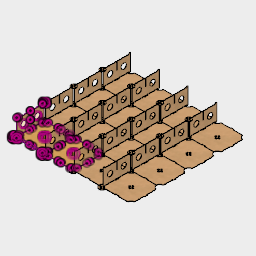
Mirobot_Labyrinth (Autodesk Fusion 360 design; units mm, degrees)
Autodesk Fusion 360 part; units mm, degrees
sketch "Sketch1" plane through (0, 0, 0) normal (0, 1, 0) x (1, 0, 0)
  line L0 (251.5519, -328.5135) -> (251.5519, -318.5135)
  line L1 (251.5519, -318.5135) -> (246.5519, -318.5135)
  line L2 (251.5519, -148.5135) -> (251.5519, -158.5135)
  line L3 (251.5519, -158.5135) -> (246.5519, -158.5135)
  line L4 (140.5519, -148.5135) -> (140.5519, -158.5135)
  line L5 (140.5519, -158.5135) -> (146.5519, -158.5135)
  line L6 (140.5519, -328.5135) -> (140.5519, -318.5135)
  line L7 (146.5519, -318.5135) -> (140.5519, -318.5135)
  line L8 (146.5519, -158.5135) -> (146.5519, -237.0135)
  line L9 (246.5519, -318.5135) -> (246.5519, -158.5135)
  circle A0 centre (166.0327, -110.4808) radius 17.5
  line L10 (251.5519, -328.5135) -> (140.5519, -328.5135)
  line L11 (140.5519, -148.5135) -> (251.5519, -148.5135)
  line L12 (161.0327, -108.9808) -> (161.0327, -111.9808)
  line L13 (161.0327, -111.9808) -> (151.0327, -111.9808)
  line L14 (151.0327, -111.9808) -> (151.0327, -108.9808)
  line L15 (151.0327, -108.9808) -> (161.0327, -108.9808)
  line L16 (167.5327, -125.4808) -> (164.5327, -125.4808)
  line L17 (164.5327, -125.4808) -> (164.5327, -115.4808)
  line L18 (167.5327, -115.4808) -> (167.5327, -125.4808)
  line L19 (164.5327, -115.4808) -> (167.5327, -115.4808)
  line L20 (181.0327, -108.9808) -> (181.0327, -111.9808)
  line L21 (181.0327, -111.9808) -> (171.0327, -111.9808)
  line L22 (171.0327, -108.9808) -> (181.0327, -108.9808)
  line L23 (171.0327, -111.9808) -> (171.0327, -108.9808)
  line L24 (164.5327, -95.4808) -> (167.5327, -95.4808)
  line L25 (167.5327, -95.4808) -> (167.5327, -105.4808)
  line L26 (164.5327, -105.4808) -> (164.5327, -95.4808)
  line L27 (167.5327, -105.4808) -> (164.5327, -105.4808)
  circle A1 centre (473.7067, -121) radius 5.0194
  circle A2 centre (463.7296, -110.8358) radius 5
  circle A3 centre (453.7523, -121) radius 5
  circle A4 centre (463.7296, -130.8358) radius 5
  circle A5 centre (663.7067, -121) radius 5.0194
  circle A6 centre (653.7296, -110.8358) radius 5
  circle A7 centre (643.7523, -121) radius 5
  circle A8 centre (653.7296, -130.8358) radius 5
  circle A9 centre (473.7067, 69) radius 5.0194
  circle A10 centre (463.7296, 79.1642) radius 5
  circle A11 centre (453.7523, 69) radius 5
  circle A12 centre (463.7296, 59.1642) radius 5
  circle A13 centre (663.7067, 69) radius 5.0194
  circle A14 centre (653.7296, 79.1642) radius 5
  circle A15 centre (643.7523, 69) radius 5
  circle A16 centre (653.7296, 59.1642) radius 5
  line L28 (443.2442, 139.3735) -> (443.2442, 139.3735)
  line L29 (436.89, 127.8892) -> (266.89, 127.8892)
  line L30 (259.39, 135.3765) -> (259.39, 135.3765)
  line L31 (266.89, 142.8892) -> (436.89, 142.8892)
  circle A17 centre (436.89, 135.3892) radius 5
  arc A18 (266.89, 142.8892) -> (259.39, 135.3765) centre (266.89, 135.3892) ccw
  arc A19 (259.39, 135.3765) -> (266.89, 127.8892) centre (266.89, 135.3892) ccw
  circle A20 centre (266.89, 135.3892) radius 5
  line L32 (453.7523, -121) -> (473.7067, -121) construction
  line L33 (463.7296, -110.8358) -> (463.7296, -130.8358) construction
  circle A21 centre (463.7295, -121) radius 25 construction
  line L34 (463.7295, -121) -> (463.7295, -146) construction
  line L35 (463.7295, -121) -> (488.7295, -121) construction
  line L36 (463.7295, -121) -> (438.7295, -121) construction
  line L37 (463.7295, -121) -> (463.7295, -96) construction
  line L38 (643.7523, -121) -> (663.7067, -121) construction
  line L39 (653.7296, -110.8358) -> (653.7296, -130.8358) construction
  circle A22 centre (653.7295, -121) radius 25 construction
  line L40 (453.7523, 69) -> (473.7067, 69) construction
  line L41 (463.7296, 79.1642) -> (463.7296, 59.1642) construction
  circle A23 centre (463.7295, 69) radius 25 construction
  line L42 (643.7523, 69) -> (663.7067, 69) construction
  line L43 (653.7296, 59.1642) -> (653.7296, 79.1642) construction
  circle A24 centre (653.7296, 69.1642) radius 25 construction
  line L44 (457.4795, -102.25) -> (461.2974, -102.25) construction
  line L45 (444.9795, -114.75) -> (449.7421, -114.75) construction
  line L46 (444.9795, -127.25) -> (440.1499, -128.5441)
  line L47 (456.1854, -144.5796) -> (440.1499, -128.5441)
  line L48 (457.4795, -139.75) -> (456.1854, -144.5796)
  line L49 (469.9795, -139.75) -> (471.2736, -144.5796)
  line L50 (487.3091, -128.5441) -> (471.2736, -144.5796)
  line L51 (482.4795, -127.25) -> (487.3091, -128.5441)
  line L52 (647.4795, -102.25) -> (646.1854, -97.4204)
  line L53 (630.1499, -113.4559) -> (646.1854, -97.4204)
  line L54 (634.9795, -114.75) -> (630.1499, -113.4559)
  line L55 (634.9795, -114.75) -> (628.7295, -121)
  line L56 (647.4799, 50.25) -> (646.1858, 45.4204)
  line L57 (646.1858, 45.4204) -> (630.1503, 61.4559)
  line L58 (634.9799, 62.75) -> (630.1503, 61.4559)
  line L59 (440.1499, -113.4559) -> (456.1854, -97.4204)
  line L60 (487.3091, 61.4559) -> (471.2736, 45.4204)
  line L61 (482.4795, 62.75) -> (487.3091, 61.4559)
  line L62 (482.4795, 62.75) -> (488.7295, 69)
  line L63 (469.9795, 50.25) -> (471.2736, 45.4204)
  line L64 (463.7293, -17.1612) -> (463.7295, 44)
  line L65 (463.7293, -17.1612) -> (468.0594, -14.6612)
  line L66 (468.0594, -14.6612) -> (468.0594, -37.3388)
  line L67 (463.7293, -34.8388) -> (468.0594, -37.3388)
  line L68 (463.7293, -34.8388) -> (463.729, -96)
  line L69 (653.7293, -34.8388) -> (653.729, -96)
  line L70 (653.7293, -34.8388) -> (658.0594, -37.3388)
  line L71 (658.0594, -14.6612) -> (658.0594, -37.3388)
  line L72 (653.7293, -17.1612) -> (658.0594, -14.6612)
  line L73 (653.7293, -17.1612) -> (653.7295, 44)
  line L74 (567.5683, -121.0002) -> (570.0683, -116.6701)
  line L75 (547.3907, -116.6701) -> (570.0683, -116.6701)
  line L76 (549.8907, -121.0002) -> (547.3907, -116.6701)
  line L77 (567.5683, 68.9998) -> (628.7295, 68.9996)
  line L78 (547.3907, 73.3299) -> (570.0683, 73.3299)
  line L79 (549.8907, 68.9998) -> (547.3907, 73.3299)
  line L80 (567.5683, 68.9998) -> (570.0683, 73.3299)
  line L81 (549.8907, 68.9998) -> (488.7295, 69)
  line L82 (628.7295, -121) -> (567.5683, -121.0002)
  line L83 (549.8907, -121.0002) -> (488.7295, -121)
  line L84 (469.9795, -139.75) -> (463.7295, -146)
  line L85 (482.4795, -127.25) -> (488.7295, -121)
  line L86 (457.4795, -139.75) -> (463.7295, -146)
  line L87 (444.9795, -127.25) -> (438.7295, -121)
  line L88 (438.7295, -121) -> (444.9795, -114.75)
  line L89 (444.9795, -114.75) -> (440.1499, -113.4559)
  line L90 (457.4795, -102.25) -> (456.1854, -97.4204)
  line L91 (463.729, -96) -> (457.4795, -102.25)
  line L92 (463.7295, 44) -> (469.9795, 50.25)
  line L93 (634.9799, 62.75) -> (628.7295, 68.9996)
  line L94 (653.7295, 44) -> (647.4799, 50.25)
  line L95 (653.729, -96) -> (647.4795, -102.25)
  arc A25 (436.89, 127.8892) -> (436.89, 142.8892) centre (436.89, 135.3892) ccw
  line L96 (146.5519, -240.0135) -> (146.5519, -318.5135)
  line L97 (196.5519, -240.0135) -> (146.5519, -240.0135)
  line L98 (196.5519, -237.0135) -> (146.5519, -237.0135)
  line L99 (196.5519, -237.0135) -> (196.5519, -240.0135)
  line L100 (198.0519, -178.5135) -> (198.0519, -188.5135)
  line L101 (195.0519, -188.5135) -> (195.0519, -178.5135)
  line L102 (191.5519, -192.0135) -> (191.5519, -195.0135)
  line L103 (211.5519, -192.0135) -> (211.5519, -195.0135)
  line L104 (191.5519, -195.0135) -> (181.5519, -195.0135)
  line L105 (195.0519, -208.5135) -> (195.0519, -198.5135)
  line L106 (198.0519, -198.5135) -> (198.0519, -208.5135)
  line L107 (198.0519, -208.5135) -> (195.0519, -208.5135)
  circle A26 centre (196.5519, -193.5135) radius 17.5
  line L108 (181.5519, -195.0135) -> (181.5519, -192.0135)
  line L109 (195.0519, -198.5135) -> (198.0519, -198.5135)
  line L110 (195.0519, -178.5135) -> (198.0519, -178.5135)
  line L111 (211.5519, -195.0135) -> (201.5519, -195.0135)
  line L112 (181.5519, -192.0135) -> (191.5519, -192.0135)
  line L113 (201.5519, -195.0135) -> (201.5519, -192.0135)
  line L114 (198.0519, -188.5135) -> (195.0519, -188.5135)
  line L115 (201.5519, -192.0135) -> (211.5519, -192.0135)
  line L116 (246.5519, -238.5135) -> (146.5519, -238.5135) construction
  circle A27 centre (196.5519, -283.5135) radius 17.5
  line L117 (201.5519, -285.0135) -> (211.5519, -285.0135)
  line L118 (211.5519, -285.0135) -> (211.5519, -282.0135)
  line L119 (201.5519, -282.0135) -> (201.5519, -285.0135)
  line L120 (211.5519, -282.0135) -> (201.5519, -282.0135)
  line L121 (195.0519, -298.5135) -> (198.0519, -298.5135)
  line L122 (198.0519, -298.5135) -> (198.0519, -288.5135)
  line L123 (195.0519, -288.5135) -> (195.0519, -298.5135)
  line L124 (198.0519, -288.5135) -> (195.0519, -288.5135)
  line L125 (181.5519, -282.0135) -> (181.5519, -285.0135)
  line L126 (181.5519, -285.0135) -> (191.5519, -285.0135)
  line L127 (191.5519, -282.0135) -> (181.5519, -282.0135)
  line L128 (191.5519, -285.0135) -> (191.5519, -282.0135)
  line L129 (198.0519, -268.5135) -> (195.0519, -268.5135)
  line L130 (195.0519, -268.5135) -> (195.0519, -278.5135)
  line L131 (198.0519, -278.5135) -> (198.0519, -268.5135)
  line L132 (195.0519, -278.5135) -> (198.0519, -278.5135)
  line L133 (463.7295, -121) -> (653.7296, 69.1642) construction
  line L134 (653.7295, -121) -> (463.7295, 69) construction
  circle A28 centre (568.7067, -26) radius 5.0194
  circle A29 centre (558.7296, -35.8358) radius 5
  circle A30 centre (548.7523, -26) radius 5
  circle A31 centre (558.7296, -15.8358) radius 5
  dimension "d4" = 10
  dimension "d6" = 10
  dimension "d7" = 10
  dimension "d8" = 3
  dimension "d11" = 180
  dimension "d12" = 100
  dimension "d34" = 5
  dimension "d50" = 10
  dimension "d53" = 10
  dimension "d66" = 6
  dimension "d80" = 50
  dimension "d83" = 50
  dimension "d85" = 50
  dimension "d87" = 50
  dimension "d109" = 170
  dimension "d113" = 170
  dimension "d124" = 111
  constraint perpendicular L12 L13
  constraint parallel L12 L14
  constraint parallel L13 L15
  constraint tangent L31 A18
  constraint tangent L29 A19
  constraint concentric A19 A20
  constraint horizontal L32
  constraint vertical L33
  constraint midpoint L32
  constraint coincident A21
  constraint perpendicular L32 L34
  constraint coincident A21 origin
  constraint perpendicular L33 L35
  constraint parallel L32 L36
  constraint parallel L33 L37
  constraint horizontal L38
  constraint midpoint L38
  constraint horizontal L40
  constraint perpendicular L40 L41
  constraint midpoint L40
  constraint horizontal L42
  constraint midpoint L43
  constraint horizontal L44
  constraint horizontal L45
  constraint perpendicular L84 L86
  constraint perpendicular L87 L88
  constraint vertical L9
  constraint horizontal L10
  constraint vertical L0
  constraint vertical L2
  constraint horizontal L3
  constraint horizontal L5
  constraint collinear L3 L5
  constraint collinear L1 L7
  constraint horizontal L29
  constraint perpendicular L96 L97
  constraint perpendicular L8 L98
  constraint perpendicular L97 L99
  constraint midpoint L9
  constraint perpendicular L9 L116
  constraint midpoint L134 origin
  measures "d11" distance of L10 L11
  measures "d12" distance of L8 L9
  measures "d50" diameter of A17
  measures "d53" diameter of A20
  measures "d66" distance of L4 L8
  measures "d80" diameter of A21
  measures "d83" diameter of A22
  measures "d85" diameter of A23
  measures "d87" diameter of A24
extrude "Extrude1" add sketch "Sketch1" along normal blind 3 contours L0 L1 L2 L3 L4 L5 L6 L7 L8 L9 L10 L11 L96 L97 L98 L99 | A0 | L29 L31 A18 A19 A25 | L46 L47 L48 L49 L50 L51 L52 L53 L54 L55 L56 L57 L58 L59 L60 L61 L62 L63 L64 L65 L66 L67 L68 L69 L70 L71 L72 L73 L74 L75 L76 L77 L78 L79 L80 L81 L82 L83 L84 L85 L86 L87 L88 L89 L90 L91 L92 L93 L94 L95 makes body 1 at (169.9494, 0, 122.1993) makes body 2 at (235.7186, 0, 223.5135) makes body 3 at (624.1003, 0, 53.8911) makes body 4 at (379.0016, 0, -129.2555)
move_body "MoveBody1" bodies 3 to x (1, 0, 0) y (0, 1, 0) z (0, 0, 1) at (-82.5386, 0, 153.1726)
pattern_linear "R-Pattern1" count 4 spacing 190 along (1, 0, 0) count 4 spacing 190 along (0, 0, -1) of bodies 3 makes body 5 at (731.5617, 0, 207.0637) makes body 6 at (921.5617, 0, 207.0637) makes body 7 at (1111.5617, 0, 207.0637) makes body 8 at (541.5617, 0, 17.0637) makes body 9 at (731.5617, 0, 17.0637) makes body 10 at (921.5617, 0, 17.0637) makes body 11 at (1111.5617, 0, 17.0637) makes body 12 at (541.5617, 0, -172.9363) makes body 13 at (731.5617, 0, -172.9363) makes body 14 at (921.5617, 0, -172.9363) makes body 15 at (1111.5617, 0, -172.9363) makes body 16 at (541.5617, 0, -362.9363) makes body 17 at (731.5617, 0, -362.9363) makes body 18 at (921.5617, 0, -362.9363) makes body 19 at (1111.5617, 0, -362.9363)
move_body "MoveBody2" bodies 4 to x (1, 0, 0) y (0, 1, 0) z (0, 0, 1) at (132.574, 0, 554.7873)
move_body "MoveBody3" bodies 2 to x (0, 1, 0) y (-1, 0, 0) z (0, 0, 1) at (253.0519, -248.5519, 0)
move_body "MoveBody4" bodies 2 to x (1, 0, 0) y (0, 0, 1) z (0, -1, 0) at (141.1162, 321.5135, 380.1726)
move_body "MoveBody5" bodies 2 to x (1, 0, 0) y (0, 0, -1) z (0, 1, 0) at (0, -271.1726, 457.1726)
move_body "MoveBody6" bodies 2 to x (1, 0, 0) y (0, 1, 0) z (0, 0, 1) at (-10.6592, 0, -193.683)
move_body "MoveBody7" bodies 2 to x (1, 0, 0) y (0, -1, 0) z (0, 0, -1) at (-1, 112, 338.9791)
move_body "MoveBody8" bodies 2 to x (1, 0, 0) y (0, 1, 0) z (0, 0, 1) at (0, 0, 20)
move_body "MoveBody9" bodies 2 to x (1, 0, 0.000003) y (0, 1, 0) z (-0.000003, 0, 1) at (1.6823, 0, -0.0013)
move_body "MoveBody10" bodies 2 to x (1, 0, 0) y (0, 1, 0) z (0, 0, 1) at (0, 0, 5.6829)
move_body "MoveBody11" bodies 2 to x (1, 0, 0) y (0, 1, 0) z (0, 0, 1) at (0, 0, -5.164)
move_body "MoveBody12" bodies 2 to x (1, 0, 0) y (0, 1, 0) z (0, 0, 1) at (-1.5, 0, 0)
pattern_linear "R-Pattern2" count 4 spacing 190 along (0, 0, -1) count 4 spacing 190 along (1, 0, 0) of bodies 2 makes body 20 at (382.6907, 15.8333, -25.9915) makes body 21 at (382.6907, 15.8333, -215.9915) makes body 22 at (382.6907, 15.8333, -405.9915) makes body 23 at (572.6907, 15.8333, 164.0085) makes body 24 at (572.6907, 15.8333, -25.9915) makes body 25 at (572.6907, 15.8333, -215.9915) makes body 26 at (572.6907, 15.8333, -405.9915) makes body 27 at (762.6907, 15.8333, 164.0085) makes body 28 at (762.6907, 15.8333, -25.9915) makes body 29 at (762.6907, 15.8333, -215.9915) makes body 30 at (762.6907, 15.8333, -405.9915) makes body 31 at (952.6907, 15.8333, 164.0085) makes body 32 at (952.6907, 15.8333, -25.9915) makes body 33 at (952.6907, 15.8333, -215.9915) makes body 34 at (952.6907, 15.8333, -405.9915)
move_body "MoveBody13" bodies 4 to x (1, 0, 0) y (0, 1, 0) z (0, 0, 1) at (-8.2959, 3, -145.2256)
sketch "Sketch3" plane through (0, 0, 0) normal (0, 1, 0) x (1, 0, 0)
  line L0 (50, -100) -> (50, -94)
  line L1 (50, -94) -> (60, -94)
  line L2 (60, -94) -> (60, -100)
  line L3 (60, -100) -> (63, -100)
  line L4 (63, -100) -> (63, -103)
  line L5 (63, -103) -> (47, -103)
  line L6 (47, -103) -> (47, -100)
  line L7 (47, -100) -> (50, -100)
  dimension "d114" = 3
  dimension "d115" = 3
  dimension "d116" = 16
  constraint horizontal L5
  constraint vertical L4
  constraint horizontal L3
  constraint vertical L2
  constraint vertical L0
  constraint horizontal L7
  constraint horizontal L1
  constraint vertical L6
extrude "Extrude2" add sketch "Sketch3" along normal blind 3 separate body makes body 35
move_body "MoveBody14" bodies 35 to x (1, 0, 0) y (0, 1, 0) z (0, 0, 1) at (349.6709, 0, 195.1812)
move_body "MoveBody15" bodies 35 to x (1, 0, 0) y (0, 0, -1) z (0, 1, 0) at (-13.5028, -289.1812, 275.6726)
move_body "MoveBody16" bodies 1 to x (1, 0, 0.000003) y (0.000003, 0, -1) z (0, 1, 0) at (203.6582, -2.9808, 97.0079)
move_body "MoveBody17" bodies 1 to x (1, 0.000003, 0.000003) y (-0.000003, 0, 1) z (0.000003, -1, 0) at (0, 200.0072, -10.4928)
move_body "MoveBody18" bodies 1 to x (1, 0, 0) y (0, 1, 0) z (0, 0, 1) at (11.5, 3, -13)
move_body "MoveBody19" bodies 1 to x (1, 0, 0) y (0, 1, 0) z (0, 0, 1) at (0, -3, 0)
pattern_linear "R-Pattern3" count 4 spacing 190 along (1, 0, 0) count 3 spacing 190 along (0, 0, -1) of bodies 1 makes body 36 at (575.1077, 106, 72.29) makes body 37 at (765.1077, 106, 72.29) makes body 38 at (955.1077, 106, 72.29) makes body 39 at (377.2744, 103, -117.71) makes body 40 at (575.1077, 106, -117.71) makes body 41 at (765.1077, 106, -117.71) makes body 42 at (955.1077, 106, -117.71) makes body 43 at (377.2744, 103, -307.71) makes body 44 at (571.691, 106, -295.3248) makes body 45 at (761.691, 106, -295.3248) makes body 46 at (951.691, 106, -295.3248)
copy_body "Body->Comp1" bodies 4 removing the originals makes body 47 in component "Rail"
copy_body "Body->Comp2" bodies 3 removing the originals makes body 48 in component "FloorPlate"
copy_body "Body->Comp3" bodies 1 removing the originals makes body 49 in component "WallConnector"
copy_body "Body->Comp4" bodies 2 removing the originals makes body 50 in component "Wall"
copy_body "Body->Comp5" bodies 35 removing the originals makes body 51 in component "RailPin"
sketch "Floor" plane through (0, 3, 0) normal (0, 1, 0) x (-1, 0, 0)
  circle A0 centre (-381.191, 264.0084) radius 5
  circle A1 centre (-381.191, 284.0084) radius 5
  circle A2 centre (-391.1681, 274.1726) radius 5.0194
  circle A3 centre (-371.2137, 274.1726) radius 5
  line L0 (-571.1907, 188.0114) -> (-575.5208, 190.5114)
  line L1 (-575.5208, 190.5114) -> (-575.5208, 167.8337)
  line L2 (-575.5208, 167.8337) -> (-571.1907, 170.3337)
  line L3 (-571.1907, 170.3337) -> (-571.1909, 109.1726)
  line L4 (-571.1909, 109.1726) -> (-564.9413, 102.9226)
  line L5 (-564.9413, 102.9226) -> (-563.6473, 107.7522)
  line L6 (-563.6473, 107.7522) -> (-547.6117, 91.7167)
  line L7 (-547.6117, 91.7167) -> (-552.4413, 90.4226)
  line L8 (-552.4413, 90.4226) -> (-546.1909, 84.173)
  line L9 (-546.1909, 84.173) -> (-485.0297, 84.1728)
  line L10 (-485.0297, 84.1728) -> (-487.5297, 79.8427)
  line L11 (-487.5297, 79.8427) -> (-464.8521, 79.8427)
  line L12 (-464.8521, 79.8427) -> (-467.3521, 84.1728)
  line L13 (-467.3521, 84.1728) -> (-406.1909, 84.1726)
  line L14 (-406.1909, 84.1726) -> (-399.9409, 90.4226)
  line L15 (-399.9409, 90.4226) -> (-404.7705, 91.7167)
  line L16 (-404.7705, 91.7167) -> (-388.735, 107.7522)
  line L17 (-388.735, 107.7522) -> (-387.4409, 102.9226)
  line L18 (-387.4409, 102.9226) -> (-381.1909, 109.1726)
  line L19 (-381.1909, 109.1726) -> (-381.1907, 170.3337)
  line L20 (-381.1907, 170.3337) -> (-385.5208, 167.8337)
  line L21 (-385.5208, 167.8337) -> (-385.5208, 190.5114)
  line L22 (-385.5208, 190.5114) -> (-381.1907, 188.0114)
  line L23 (-381.1907, 188.0114) -> (-381.1905, 249.1726)
  line L24 (-381.1905, 249.1726) -> (-374.9409, 255.4226)
  line L25 (-374.9409, 255.4226) -> (-373.6468, 250.593)
  line L26 (-373.6468, 250.593) -> (-357.6113, 266.6285)
  line L27 (-357.6113, 266.6285) -> (-362.4409, 267.9226)
  line L28 (-362.4409, 267.9226) -> (-356.1909, 274.1726)
  line L29 (-356.1909, 274.1726) -> (-362.4409, 280.4226)
  line L30 (-362.4409, 280.4226) -> (-357.6113, 281.7167)
  line L31 (-357.6113, 281.7167) -> (-373.6468, 297.7522)
  line L32 (-373.6468, 297.7522) -> (-374.9409, 292.9226)
  line L33 (-374.9409, 292.9226) -> (-381.1909, 299.1726)
  line L34 (-381.1909, 299.1726) -> (-387.4409, 292.9226)
  line L35 (-387.4409, 292.9226) -> (-388.735, 297.7522)
  line L36 (-388.735, 297.7522) -> (-404.7705, 281.7167)
  line L37 (-404.7705, 281.7167) -> (-399.9409, 280.4226)
  line L38 (-399.9409, 280.4226) -> (-406.1909, 274.1726)
  line L39 (-406.1909, 274.1726) -> (-467.3521, 274.1728)
  line L40 (-467.3521, 274.1728) -> (-464.8521, 269.8427)
  line L41 (-464.8521, 269.8427) -> (-487.5297, 269.8427)
  line L42 (-487.5297, 269.8427) -> (-485.0297, 274.1728)
  line L43 (-485.0297, 274.1728) -> (-546.1909, 274.1726)
  line L44 (-546.1909, 274.1726) -> (-552.4409, 267.9226)
  line L45 (-552.4409, 267.9226) -> (-547.6113, 266.6285)
  line L46 (-547.6113, 266.6285) -> (-563.6468, 250.593)
  line L47 (-563.6468, 250.593) -> (-564.9409, 255.4226)
  line L48 (-564.9409, 255.4226) -> (-571.1905, 249.1726)
  line L49 (-571.1905, 249.1726) -> (-571.1907, 188.0114)
  line L50 (-546.1909, 84.173) -> (-485.0297, 84.1728)
  circle A4 centre (-381.191, 264.0084) radius 5
  circle A5 centre (-381.191, 284.0084) radius 5
  circle A6 centre (-391.1681, 274.1726) radius 5.0194
  circle A7 centre (-371.2137, 274.1726) radius 5
  line L51 (-575.5208, 190.5114) -> (-571.1907, 188.0114)
  line L52 (-571.1907, 188.0114) -> (-571.1905, 249.1726)
  line L53 (-571.1905, 249.1726) -> (-564.9409, 255.4226)
  line L54 (-564.9409, 255.4226) -> (-563.6468, 250.593)
  line L55 (-563.6468, 250.593) -> (-547.6113, 266.6285)
  line L56 (-547.6113, 266.6285) -> (-552.4409, 267.9226)
  line L57 (-552.4409, 267.9226) -> (-546.1909, 274.1726)
  line L58 (-546.1909, 274.1726) -> (-485.0297, 274.1728)
  line L59 (-485.0297, 274.1728) -> (-487.5297, 269.8427)
  line L60 (-487.5297, 269.8427) -> (-464.8521, 269.8427)
  line L61 (-464.8521, 269.8427) -> (-467.3521, 274.1728)
  line L62 (-467.3521, 274.1728) -> (-406.1909, 274.1726)
  line L63 (-406.1909, 274.1726) -> (-399.9409, 280.4226)
  line L64 (-399.9409, 280.4226) -> (-404.7705, 281.7167)
  line L65 (-404.7705, 281.7167) -> (-388.735, 297.7522)
  line L66 (-388.735, 297.7522) -> (-387.4409, 292.9226)
  line L67 (-387.4409, 292.9226) -> (-381.1909, 299.1726)
  line L68 (-381.1909, 299.1726) -> (-374.9409, 292.9226)
  line L69 (-374.9409, 292.9226) -> (-373.6468, 297.7522)
  line L70 (-373.6468, 297.7522) -> (-357.6113, 281.7167)
  line L71 (-357.6113, 281.7167) -> (-362.4409, 280.4226)
  line L72 (-362.4409, 280.4226) -> (-356.1909, 274.1726)
  line L73 (-356.1909, 274.1726) -> (-362.4409, 267.9226)
  line L74 (-362.4409, 267.9226) -> (-357.6113, 266.6285)
  line L75 (-357.6113, 266.6285) -> (-373.6468, 250.593)
  line L76 (-373.6468, 250.593) -> (-374.9409, 255.4226)
  line L77 (-374.9409, 255.4226) -> (-381.1905, 249.1726)
  line L78 (-381.1905, 249.1726) -> (-381.1907, 188.0114)
  line L79 (-381.1907, 188.0114) -> (-385.5208, 190.5114)
  line L80 (-385.5208, 190.5114) -> (-385.5208, 167.8337)
  line L81 (-385.5208, 167.8337) -> (-381.1907, 170.3337)
  line L82 (-381.1907, 170.3337) -> (-381.1909, 109.1726)
  line L83 (-381.1909, 109.1726) -> (-387.4409, 102.9226)
  line L84 (-387.4409, 102.9226) -> (-388.735, 107.7522)
  line L85 (-388.735, 107.7522) -> (-404.7705, 91.7167)
  line L86 (-404.7705, 91.7167) -> (-399.9409, 90.4226)
  line L87 (-399.9409, 90.4226) -> (-406.1909, 84.1726)
  line L88 (-406.1909, 84.1726) -> (-467.3521, 84.1728)
  line L89 (-467.3521, 84.1728) -> (-464.8521, 79.8427)
  line L90 (-464.8521, 79.8427) -> (-487.5297, 79.8427)
  line L91 (-487.5297, 79.8427) -> (-485.0297, 84.1728)
  line L92 (-485.0297, 84.1728) -> (-546.1909, 84.173)
  line L93 (-546.1909, 84.173) -> (-552.4413, 90.4226)
  line L94 (-552.4413, 90.4226) -> (-547.6117, 91.7167)
  line L95 (-547.6117, 91.7167) -> (-563.6473, 107.7522)
  line L96 (-563.6473, 107.7522) -> (-564.9413, 102.9226)
  line L97 (-564.9413, 102.9226) -> (-571.1909, 109.1726)
  line L98 (-571.1909, 109.1726) -> (-571.1907, 170.3337)
  line L99 (-571.1907, 170.3337) -> (-575.5208, 167.8337)
  line L100 (-575.5208, 167.8337) -> (-575.5208, 190.5114)
  circle A8 centre (-571.191, 264.0084) radius 5
  circle A9 centre (-571.191, 284.0084) radius 5
  circle A10 centre (-581.1681, 274.1726) radius 5.0194
  circle A11 centre (-561.2137, 274.1726) radius 5
  line L101 (-761.1907, 188.0114) -> (-765.5208, 190.5114)
  line L102 (-765.5208, 190.5114) -> (-765.5208, 167.8337)
  line L103 (-765.5208, 167.8337) -> (-761.1907, 170.3337)
  line L104 (-761.1907, 170.3337) -> (-761.1909, 109.1726)
  line L105 (-761.1909, 109.1726) -> (-754.9413, 102.9226)
  line L106 (-754.9413, 102.9226) -> (-753.6473, 107.7522)
  line L107 (-753.6473, 107.7522) -> (-737.6117, 91.7167)
  line L108 (-737.6117, 91.7167) -> (-742.4413, 90.4226)
  line L109 (-742.4413, 90.4226) -> (-736.1909, 84.173)
  line L110 (-736.1909, 84.173) -> (-675.0297, 84.1728)
  line L111 (-675.0297, 84.1728) -> (-677.5297, 79.8427)
  line L112 (-677.5297, 79.8427) -> (-654.8521, 79.8427)
  line L113 (-654.8521, 79.8427) -> (-657.3521, 84.1728)
  line L114 (-657.3521, 84.1728) -> (-596.1909, 84.1726)
  line L115 (-596.1909, 84.1726) -> (-589.9409, 90.4226)
  line L116 (-589.9409, 90.4226) -> (-594.7705, 91.7167)
  line L117 (-594.7705, 91.7167) -> (-578.735, 107.7522)
  line L118 (-578.735, 107.7522) -> (-577.4409, 102.9226)
  line L119 (-577.4409, 102.9226) -> (-571.1909, 109.1726)
  line L120 (-571.1909, 109.1726) -> (-571.1907, 170.3337)
  line L121 (-571.1907, 170.3337) -> (-575.5208, 167.8337)
  line L122 (-575.5208, 167.8337) -> (-575.5208, 190.5114)
  line L123 (-575.5208, 190.5114) -> (-571.1907, 188.0114)
  line L124 (-571.1907, 188.0114) -> (-571.1905, 249.1726)
  line L125 (-571.1905, 249.1726) -> (-564.9409, 255.4226)
  line L126 (-564.9409, 255.4226) -> (-563.6468, 250.593)
  line L127 (-563.6468, 250.593) -> (-547.6113, 266.6285)
  line L128 (-547.6113, 266.6285) -> (-552.4409, 267.9226)
  line L129 (-552.4409, 267.9226) -> (-546.1909, 274.1726)
  line L130 (-546.1909, 274.1726) -> (-552.4409, 280.4226)
  line L131 (-552.4409, 280.4226) -> (-547.6113, 281.7167)
  line L132 (-547.6113, 281.7167) -> (-563.6468, 297.7522)
  line L133 (-563.6468, 297.7522) -> (-564.9409, 292.9226)
  line L134 (-564.9409, 292.9226) -> (-571.1909, 299.1726)
  line L135 (-571.1909, 299.1726) -> (-577.4409, 292.9226)
  line L136 (-577.4409, 292.9226) -> (-578.735, 297.7522)
  line L137 (-578.735, 297.7522) -> (-594.7705, 281.7167)
  line L138 (-594.7705, 281.7167) -> (-589.9409, 280.4226)
  line L139 (-589.9409, 280.4226) -> (-596.1909, 274.1726)
  line L140 (-596.1909, 274.1726) -> (-657.3521, 274.1728)
  line L141 (-657.3521, 274.1728) -> (-654.8521, 269.8427)
  line L142 (-654.8521, 269.8427) -> (-677.5297, 269.8427)
  line L143 (-677.5297, 269.8427) -> (-675.0297, 274.1728)
  line L144 (-675.0297, 274.1728) -> (-736.1909, 274.1726)
  line L145 (-736.1909, 274.1726) -> (-742.4409, 267.9226)
  line L146 (-742.4409, 267.9226) -> (-737.6113, 266.6285)
  line L147 (-737.6113, 266.6285) -> (-753.6468, 250.593)
  line L148 (-753.6468, 250.593) -> (-754.9409, 255.4226)
  line L149 (-754.9409, 255.4226) -> (-761.1905, 249.1726)
  line L150 (-761.1905, 249.1726) -> (-761.1907, 188.0114)
  circle A12 centre (-486.1681, 179.1726) radius 5.0194
  circle A13 centre (-466.2137, 179.1726) radius 5
  circle A14 centre (-476.191, 169.0084) radius 5
  circle A15 centre (-476.191, 189.0084) radius 5
  circle A16 centre (-486.1681, 179.1726) radius 5.0194
  circle A17 centre (-466.2137, 179.1726) radius 5
  circle A18 centre (-476.191, 169.0084) radius 5
  circle A19 centre (-476.191, 189.0084) radius 5
  circle A20 centre (-676.1681, 179.1726) radius 5.0194
  circle A21 centre (-656.2137, 179.1726) radius 5
  circle A22 centre (-666.191, 169.0084) radius 5
  circle A23 centre (-666.191, 189.0084) radius 5
sketch "Wall" plane through (379.6913, 0, 0.0013) normal (-1, 0, -0.000003) x (-0.000003, 0, 1)
  line L0 (259.0072, 111) -> (259.0072, 105)
  line L1 (259.0072, 105) -> (180.5072, 105)
  line L2 (99.0072, 105) -> (99.0072, 111)
  line L3 (99.0072, 111) -> (89.0072, 111)
  line L4 (89.0072, 111) -> (89.0072, 0)
  line L5 (89.0072, 0) -> (99.0072, 0)
  line L6 (99.0072, 0) -> (99.0072, 5)
  line L7 (99.0072, 5) -> (259.0072, 5)
  line L8 (259.0072, 5) -> (259.0072, 0)
  line L9 (259.0072, 0) -> (269.0072, 0)
  line L10 (269.0072, 0) -> (269.0072, 111)
  line L11 (269.0072, 111) -> (259.0072, 111)
  line L12 (259.0072, 105) -> (259.0072, 111)
  line L13 (259.0072, 111) -> (269.0072, 111)
  line L14 (269.0072, 111) -> (269.0072, 0)
  line L15 (269.0072, 0) -> (259.0072, 0)
  line L16 (259.0072, 0) -> (259.0072, 5)
  line L17 (259.0072, 5) -> (99.0072, 5)
  line L18 (99.0072, 5) -> (99.0072, 0)
  line L19 (99.0072, 0) -> (89.0072, 0)
  line L20 (89.0072, 0) -> (89.0072, 111)
  line L21 (89.0072, 111) -> (99.0072, 111)
  line L22 (99.0072, 111) -> (99.0072, 105)
  line L23 (180.5072, 105) -> (259.0072, 105)
  line L24 (180.5072, 105) -> (180.5072, 55)
  line L25 (180.5072, 55) -> (177.5072, 55)
  line L26 (177.5072, 55) -> (177.5072, 105)
  line L27 (177.5072, 105) -> (99.0072, 105)
  line L28 (99.0072, 105) -> (177.5072, 105)
  line L29 (177.5072, 105) -> (177.5072, 55)
  line L30 (177.5072, 55) -> (180.5072, 55)
  line L31 (180.5072, 55) -> (180.5072, 105)
  circle A0 centre (224.0072, 55) radius 17.5
  circle A1 centre (134.0072, 55) radius 17.5
  circle A2 centre (224.0072, 55) radius 17.5
  circle A3 centre (134.0072, 55) radius 17.5
sketch "Pin" plane through (0, 0, 275.6726) normal (0, 0, 1) x (1, 0, 0)
  line L0 (383.1681, 9) -> (383.1681, 6)
  line L1 (383.1681, 6) -> (386.1681, 6)
  line L2 (386.1681, 6) -> (386.1681, 0)
  line L3 (386.1681, 0) -> (396.1681, 0)
  line L4 (396.1681, 0) -> (396.1681, 6)
  line L5 (396.1681, 6) -> (399.1681, 6)
  line L6 (399.1681, 6) -> (399.1681, 9)
  line L7 (399.1681, 9) -> (383.1681, 9)
  line L8 (383.1681, 6) -> (383.1681, 9)
  line L9 (383.1681, 9) -> (399.1681, 9)
  line L10 (399.1681, 9) -> (399.1681, 6)
  line L11 (399.1681, 6) -> (396.1681, 6)
  line L12 (396.1681, 6) -> (396.1681, 0)
  line L13 (396.1681, 0) -> (386.1681, 0)
  line L14 (386.1681, 0) -> (386.1681, 6)
  line L15 (386.1681, 6) -> (383.1681, 6)
sketch "WallConnector" plane through (0, 106, 0) normal (0, 1, 0) x (-1, 0, 0)
  line L0 (-382.691, 69.0085) -> (-382.691, 79.0085)
  line L1 (-382.691, 79.0085) -> (-379.691, 79.0085)
  line L2 (-379.691, 79.0085) -> (-379.691, 69.0085)
  line L3 (-379.691, 69.0085) -> (-382.691, 69.0085)
  line L4 (-379.6909, 99.0085) -> (-379.691, 89.0085)
  line L5 (-379.691, 89.0085) -> (-382.691, 89.0085)
  line L6 (-382.691, 89.0085) -> (-382.6909, 99.0085)
  line L7 (-382.6909, 99.0085) -> (-379.6909, 99.0085)
  line L8 (-366.191, 85.5084) -> (-366.191, 82.5084)
  line L9 (-366.191, 82.5084) -> (-376.191, 82.5085)
  line L10 (-376.191, 82.5085) -> (-376.191, 85.5085)
  line L11 (-376.191, 85.5085) -> (-366.191, 85.5084)
  line L12 (-396.191, 85.5085) -> (-386.191, 85.5085)
  line L13 (-386.191, 85.5085) -> (-386.191, 82.5085)
  line L14 (-386.191, 82.5085) -> (-396.191, 82.5085)
  line L15 (-396.191, 82.5085) -> (-396.191, 85.5085)
  circle A0 centre (-381.191, 84.0085) radius 17.5
  line L16 (-382.691, 79.0085) -> (-382.691, 69.0085)
  line L17 (-382.691, 69.0085) -> (-379.691, 69.0085)
  line L18 (-379.691, 69.0085) -> (-379.691, 79.0085)
  line L19 (-379.691, 79.0085) -> (-382.691, 79.0085)
  line L20 (-379.691, 89.0085) -> (-379.6909, 99.0085)
  line L21 (-379.6909, 99.0085) -> (-382.6909, 99.0085)
  line L22 (-382.6909, 99.0085) -> (-382.691, 89.0085)
  line L23 (-382.691, 89.0085) -> (-379.691, 89.0085)
  line L24 (-366.191, 82.5084) -> (-366.191, 85.5084)
  line L25 (-366.191, 85.5084) -> (-376.191, 85.5085)
  line L26 (-376.191, 85.5085) -> (-376.191, 82.5085)
  line L27 (-376.191, 82.5085) -> (-366.191, 82.5084)
  line L28 (-386.191, 85.5085) -> (-396.191, 85.5085)
  line L29 (-396.191, 85.5085) -> (-396.191, 82.5085)
  line L30 (-396.191, 82.5085) -> (-386.191, 82.5085)
  line L31 (-386.191, 82.5085) -> (-386.191, 85.5085)
  circle A1 centre (-381.191, 84.0085) radius 17.5
sketch "Bar" plane through (0, 6, 0) normal (0, 1, 0) x (-1, 0, 0)
  circle A0 centre (-561.1681, 274.1726) radius 5
  circle A1 centre (-391.1681, 274.1726) radius 5
  arc A2 (-391.1681, 266.6726) -> (-391.1681, 281.6726) centre (-391.1681, 274.1726) ccw
  line L0 (-391.1681, 281.6726) -> (-561.1681, 281.6726)
  arc A3 (-561.1681, 281.6726) -> (-561.1681, 266.6726) centre (-561.1681, 274.1726) ccw
  line L1 (-561.1681, 266.6726) -> (-391.1681, 266.6726)
  line L2 (-391.1681, 281.6726) -> (-561.1681, 281.6726)
  circle A4 centre (-561.1681, 274.1726) radius 5
  circle A5 centre (-391.1681, 274.1726) radius 5
  arc A6 (-391.1681, 266.6726) -> (-391.1681, 281.6726) centre (-391.1681, 274.1726) ccw
  line L3 (-391.1681, 266.6726) -> (-561.1681, 266.6726)
  arc A7 (-561.1681, 281.6726) -> (-561.1681, 266.6726) centre (-561.1681, 274.1726) ccw
  line L4 (-561.1681, 281.6726) -> (-391.1681, 281.6726)
component "Rail" placed x (1, 0, 0) y (0, 1, 0) z (0, 0, 1) at (0, 0, 0)
component "FloorPlate" placed x (1, 0, 0) y (0, 1, 0) z (0, 0, 1) at (0, 0, 0)
component "WallConnector" placed x (1, 0, 0) y (0, 1, 0) z (0, 0, 1) at (0, 0, 0)
component "Wall" placed x (1, 0, 0) y (0, 1, 0) z (0, 0, 1) at (0, 0, 0)
component "RailPin" placed x (1, 0, 0) y (0, 1, 0) z (0, 0, 1) at (0, 0, 0)
equation "d101 = ( 190 * 3 ) * 1 mm"
equation "d102 = -( 190 * 3 ) * 1 mm"
equation "d107 = ( -( 190 ) * 3 ) * 1 mm"
equation "d108 = ( 190 * 3 ) * 1 mm"
equation "d121 = ( 3 * 190 ) * 1 mm"
equation "d122 = ( -2 * 190 ) * 1 mm"
named bodies: "WallConnector", "Wall", "FloorPlate", "Rail", "FloorPlate (1)", "FloorPlate (2)", "FloorPlate (3)", "FloorPlate (4)", "FloorPlate (5)", "FloorPlate (6)", "FloorPlate (7)", "FloorPlate (8)", "FloorPlate (9)", "FloorPlate (10)", "FloorPlate (11)", "FloorPlate (12)", "FloorPlate (13)", "FloorPlate (14)", "FloorPlate (15)", "Wall (1)", "Wall (2)", "Wall (3)", "Wall (4)", "Wall (5)", "Wall (6)", "Wall (7)", "Wall (8)", "Wall (9)", "Wall (10)", "Wall (11)", "Wall (12)", "Wall (13)", "Wall (14)", "Wall (15)", "RailPin", "WallConnector (1)", "WallConnector (2)", "WallConnector (3)", "WallConnector (4)", "WallConnector (5)", "WallConnector (6)", "WallConnector (7)", "WallConnector (8)", "WallConnector (9)", "WallConnector (10)", "WallConnector (11)"
